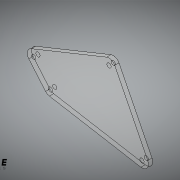
# Autodesk Inventor part: 中間外フレーム
Saved by Autodesk Inventor 2019 (Build 230136000, 136)
## iProperties
Created: 2019-09-17
Part Number: 中間外フレーム
Material: ポリカーボネート、クリア
Document SubType Name: Modeling
Designer: tanjihayato
Density: 1.2 g/cm^3
Appearance: ポリカーボネート - クリア
Author: tanjihayato
Autodesk Inventor part; units mm, degrees
ref_plane "YZ Plane" through (0, 0, 0) normal (1, 0, 0) x (0, 1, 0)
ref_plane "XZ Plane" through (0, 0, 0) normal (0, 1, 0) x (-1, 0, 0)
ref_plane "XY Plane" through (0, 0, 0) normal (0, 0, 1) x (1, 0, 0)
sketch "スケッチ2" plane through (0, 0, 0) normal (0, 0, 1) x (1, 0, 0)
  circle A0 centre (0, 0) radius 10.1 construction
  circle A1 centre (25.3202, -9.9362) radius 17.1 construction
  circle A2 centre (110.4743, -16.4118) radius 28.1 construction
  circle A3 centre (62.4131, -12.7569) radius 20.1 construction
  circle A4 centre (-21.6908, -16.4118) radius 17.1 construction
  circle A5 centre (-105.5257, -16.4118) radius 28.1 construction
  line L0 (-170.915, -81.4118) -> (490.0044, -81.4118)
  line L1 (-105.5257, -16.4118) -> (-21.6908, -16.4118) construction
  line L2 (110.4743, -16.4118) -> (25.3202, -9.9362) construction
  line L3 (110.4743, -16.4118) -> (104.1501, -0.632)
  line L4 (104.1501, -0.632) -> (95.5937, 20.7173) construction
  line L5 (95.5937, 20.7173) -> (70.4743, -10.4118) construction
  line L6 (70.4743, -10.4118) -> (110.4743, -16.4118) construction
  line L7 (-137.6819, 53.5882) -> (165.8186, 53.5882)
  line L8 (25.3202, -9.9362) -> (108.6869, 8.5882) construction
  line L9 (25.3202, -9.9362) -> (102.5386, -46.4118) construction
  line L10 (25.3202, -9.9362) -> (5.9362, 53.5882) construction
  line L11 (5.9362, 53.5882) -> (127.6431, 30.2622)
  line L12 (127.6431, 30.2622) -> (110.4743, -16.4118) construction
  line L13 (102.5386, -46.4118) -> (118.0681, 0.8329) construction
  line L14 (118.0681, 0.8329) -> (5.9362, 53.5882) construction
  line L15 (108.6869, 8.5882) -> (129.8583, 53.5882) construction
  line L16 (129.8583, 53.5882) -> (5.9362, 53.5882) construction
  line L17 (119.2726, 31.0882) -> (366.4441, 68.5882) construction
  line L18 (119.0587, 6.9252) -> (362.0213, 65.8249) construction
  line L19 (110.3034, -22.7894) -> (351.0624, 44.5537) construction
  line L20 (127.6431, 30.2622) -> (4.1927, 19.4617) construction
  circle A6 centre (80.4743, 23.124) radius 3 construction
  circle A7 centre (80.4743, 23.124) radius 1.5
  arc A8 (79.801, 27.5733) -> (76.162, 24.4099) centre (80.4743, 23.124) ccw
  circle A9 centre (70.4743, -10.4118) radius 1.5
  arc A10 (66.162, -9.1259) -> (69.4242, -14.7876) centre (70.4743, -10.4118) ccw
  circle A11 centre (150.4743, 0.5882) radius 1.5
  arc A12 (152.5623, -3.3981) -> (154.0408, 3.3323) centre (150.4743, 0.5882) ccw
  circle A13 centre (127.6431, 30.2622) radius 1.5
  arc A14 (131.2816, 32.9102) -> (126.9698, 34.7115) centre (127.6431, 30.2622) ccw
  circle A15 centre (110.4743, -16.4118) radius 5
  arc A16 (108.6075, -24.1909) -> (114.1862, -23.4986) centre (110.4743, -16.4118) ccw
  line L21 (76.162, 24.4099) -> (66.162, -9.1259)
  line L22 (69.4242, -14.7876) -> (108.6075, -24.1909)
  line L23 (114.1862, -23.4986) -> (152.5623, -3.3981)
  line L24 (154.0408, 3.3323) -> (131.2097, 33.0062)
  line L25 (126.9698, 34.7115) -> (79.801, 27.5733)
  circle A17 centre (-145.5257, 0.5882) radius 1.5
  arc A18 (-149.0922, 3.3323) -> (-147.6136, -3.3981) centre (-145.5257, 0.5882) ccw
  circle A19 centre (-105.5257, -16.4118) radius 5
  arc A20 (-109.2375, -23.4986) -> (-103.6588, -24.1909) centre (-105.5257, -16.4118) ccw
  circle A21 centre (-65.5257, -10.4118) radius 1.5
  arc A22 (-64.4756, -14.7876) -> (-61.2133, -9.1259) centre (-65.5257, -10.4118) ccw
  circle A23 centre (0, 0) radius 20.05 construction
  circle A24 centre (110.4743, -16.4118) radius 30.1 construction
  circle A25 centre (62.4131, -12.7569) radius 22.1 construction
  circle A26 centre (25.3202, -9.9362) radius 19.1 construction
  circle A27 centre (0, 0) radius 12.1 construction
  circle A28 centre (-21.6908, -16.4118) radius 19.1 construction
  circle A29 centre (-105.5257, -16.4118) radius 30.1 construction
  circle A30 centre (0, 0) radius 20.55 construction
  circle A31 centre (95.5937, 20.7173) radius 4.025 construction
  circle A32 centre (95.5937, 20.7173) radius 6.025 construction
  circle A33 centre (-75.5257, 23.124) radius 1.5
  arc A34 (-71.2133, 24.4099) -> (-74.8523, 27.5733) centre (-75.5257, 23.124) ccw
  circle A35 centre (-122.6945, 30.2622) radius 1.5
  arc A36 (-122.0212, 34.7115) -> (-126.261, 33.0062) centre (-122.6945, 30.2622) ccw
  line L26 (-126.261, 33.0062) -> (-149.0922, 3.3323)
  line L27 (-147.6136, -3.3981) -> (-109.2375, -23.4986)
  line L28 (-103.6588, -24.1909) -> (-64.4756, -14.7876)
  line L29 (-61.2133, -9.1259) -> (-71.2133, 24.4099)
  line L30 (-74.8523, 27.5733) -> (-122.0212, 34.7115)
  circle A37 centre (14, -17.4118) radius 2.2921 construction
  circle A38 centre (-14, -17.4118) radius 2.2921 construction
  circle A39 centre (-14, -17.4118) radius 14 construction
  circle A40 centre (14, -17.4118) radius 14 construction
  line L31 (-170.6512, -31.4118) -> (202.8656, -31.4118)
  line L32 (5.9362, 53.5882) -> (-38.6574, 35.6253) construction
  line L33 (5.9362, 53.5882) -> (-26.7676, 18.3503) construction
  circle A41 centre (5.9362, 53.5882) radius 1.5
  arc A42 (9.9603, 55.6024) -> (4.2549, 57.7623) centre (5.9362, 53.5882) ccw
  line L34 (-21.6908, -16.4118) -> (-99.9742, 13.5882) construction
  line L35 (-21.6908, -16.4118) -> (-101.7113, -41.4118) construction
  line L36 (9.9603, 55.6024) -> (33.1621, 9.2488)
  circle A43 centre (-47.0055, 32.2626) radius 1.5
  arc A44 (-48.6869, 36.4367) -> (-50.4404, 29.3554) centre (-47.0055, 32.2626) ccw
  line L37 (4.2549, 57.7623) -> (-48.6869, 36.4367)
  line L38 (-50.4404, 29.3554) -> (-38.6655, 15.4431)
  circle A45 centre (29.1381, 7.2346) radius 3 construction
  circle A46 centre (-84.8661, 5.2713) radius 4.5 construction
  circle A47 centre (-132.0174, -1.9813) radius 4.5 construction
  line L39 (-132.7015, 2.4664) -> (-85.5502, 9.719) construction
  arc A48 (28.3723, 2.8003) -> (33.1621, 9.2488) centre (29.1381, 7.2346) ccw
  arc A49 (-38.6655, 15.4431) -> (-35.9964, 13.9159) centre (-35.2306, 18.3503) ccw
  line L40 (-35.9964, 13.9159) -> (28.3723, 2.8003)
  circle A50 centre (-38.6574, 35.6253) radius 3 construction
  circle A51 centre (25.3202, -9.9362) radius 4.025 construction
  circle A52 centre (-21.6908, -16.4118) radius 4.025 construction
  circle A53 centre (-35.2306, 18.3503) radius 1.5
  circle A54 centre (29.1381, 7.2346) radius 1.5
  circle A55 centre (-57.813, 39.7705) radius 4.5 construction
  circle A56 centre (-99.304, 63.3152) radius 4.5 construction
  line L41 (5.9362, 53.5882) -> (-32.8159, 25.1361) construction
  circle A57 centre (-58.0056, -24.4791) radius 20.1 construction
  circle A58 centre (-58.0056, -24.4791) radius 22.1 construction
  line L42 (-53.3261, 39.4281) -> (-56.2797, 0.7243) construction
  circle A59 centre (-38.6574, 35.6253) radius 4.5
  dimension "d207" = 9
  dimension "d208" = 9
  dimension "d223" = 9
  dimension "d119" = 20.2
  dimension "d120" = 34.2
  dimension "d121" = 56.2
  dimension "d122" = 40.2
  dimension "d123" = 216
  dimension "d124" = 65
  dimension "d125" = 65
  dimension "d126" = 34.2
  dimension "d127" = 56.2
  dimension "d128" = 17
  dimension "d129" = 23
  dimension "d130" = 40
  dimension "d131" = 40
  dimension "d132" = 6
  dimension "d133" = 135
  dimension "d134" = 25
  dimension "d135" = 30
  dimension "d136" = 5
  dimension "d137" = 2
  dimension "d138" = 250
  dimension "d139" = 150
  dimension "d140" = 250
  dimension "d141" = 250
  dimension "d142" = 123.823
  dimension "d143" = 123.823
  dimension "d144" = 123.823
  dimension "d145" = 6
  dimension "d146" = 3
  dimension "d147" = 9
  dimension "d148" = 3
  dimension "d149" = 9
  dimension "d150" = 3
  dimension "d151" = 9
  dimension "d152" = 40
  dimension "d153" = 17
  dimension "d154" = 3
  dimension "d155" = 9
  dimension "d156" = 10
  dimension "d157" = 3
  dimension "d158" = 3
  dimension "d159" = 9
  dimension "d160" = 40
  dimension "d161" = 17
  dimension "d162" = 10
  dimension "d163" = 3
  dimension "d164" = 3
  dimension "d165" = 9
  dimension "d166" = 40
  dimension "d167" = 6
  dimension "d168" = 40.1
  dimension "d169" = 2
  dimension "d170" = 2
  dimension "d171" = 2
  dimension "d172" = 2
  dimension "d173" = 2
  dimension "d174" = 2
  dimension "d175" = 0.5
  dimension "d176" = 8.05
  dimension "d177" = 2
  dimension "d178" = 3
  dimension "d179" = 9
  dimension "d180" = 3
  dimension "d181" = 9
  dimension "d182" = 46.674
  constraints: 86 end point, 57 centre point, 39 tangent, 29 coincident, 29 point on circle, 11 equal length, 5 horizontal, 3 midpoint, 3 point on line, 2 equal radius, 1 collinear, 1 parallel, 1 perpendicular, 13 other
  measures "d119" diameter of A0
  measures "d120" diameter of A1
  measures "d121" diameter of A2
  measures "d122" diameter of A3
  measures "d123" distance of L1.start L2.start
  measures "d124" distance from line of L0 L2.start
  measures "d125" distance from line of L0 L1.start
  measures "d126" diameter of A4
  measures "d127" diameter of A5
  measures "d128" distance of L2.start L3.end
  measures "d129" distance of L3.end L4.end
  measures "d130" distance of L4.end L5.end
  measures "d131" horizontal distance of L5.end L2.start
  measures "d132" vertical distance of L5.end L2.start
  measures "d133" distance between parallel lines of L0 L7
  measures "d134" vertical distance of L2.start L8.end
  measures "d135" vertical distance of L9.end L2.start
  measures "d136" angle of L12 L15
  measures "d137" angle of L12 L13
  measures "d138" distance of L17.start L17.end
  measures "d139" distance from line of L0 L17.end
  measures "d140" distance of L18.start L18.end
  measures "d141" distance of L19.start L19.end
  measures "d142" angle of L15 L17
  measures "d143" angle of L12 L18
  measures "d144" angle of L13 L19
  measures "d145" diameter of A6
  measures "d146" diameter of A7
  measures "d147" diameter of A8
  measures "d148" diameter of A9
  measures "d149" diameter of A10
  measures "d150" diameter of A11
  measures "d151" diameter of A12
  measures "d152" horizontal distance of L2.start A11.centre
  measures "d153" vertical distance of L2.start A11.centre
  measures "d154" diameter of A13
  measures "d155" diameter of A14
  measures "d156" diameter of A15
  measures "d157" radial gap between concentric circles of A15 A16
  measures "d158" diameter of A17
  measures "d159" diameter of A18
  measures "d160" horizontal distance of L1.start A17.centre
  measures "d161" vertical distance of L1.start A18.centre
  measures "d162" diameter of A19
  measures "d163" radial gap between concentric circles of A19 A20
  measures "d164" diameter of A21
  measures "d165" diameter of A22
  measures "d166" horizontal distance of L1.start A21.centre
  measures "d167" vertical distance of L1.start A21.centre
  measures "d168" diameter of A23
  measures "d169" radial gap between concentric circles of A2 A24
  measures "d170" radial gap between concentric circles of A3 A25
  measures "d171" radial gap between concentric circles of A1 A26
  measures "d172" radial gap between concentric circles of A0 A27
  measures "d173" radial gap between concentric circles of A4 A28
  measures "d174" radial gap between concentric circles of A5 A29
  measures "d175" radial gap between concentric circles of A23 A30
  measures "d176" diameter of A31
  measures "d177" radial gap between concentric circles of A31 A32
  measures "d178" diameter of A33
  measures "d179" diameter of A34
  measures "d180" diameter of A35
  measures "d181" diameter of A36
  measures "d182" vertical distance of L2.start L11.end
extrude "押し出し2" add sketch "スケッチ2" along normal blind 3 contours A41 L7 L37 A42 L36 | L7 L36 L11 A41 | A59 | A41 L11 L36 A48 L40 A49 L38 A44 L37 L7
equation "\"d126\" = d120"
equation "\"d127\" = d121"
equation "\"d143\" = d142"
equation "\"d144\" = d142"
